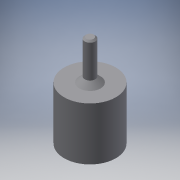
# Autodesk Inventor part: Transmission_Mount_Tester
Saved by Autodesk Inventor 2016 (Build 200138000, 138)
## iProperties
Created: 2015-07-24
Part Number: Transmission_Mount_Tester
Material: Generic
Document SubType Name: Modeling
Designer: 3DPrinterUser
Density: 1 g/cm^3
Appearance: Default
Author: 3DPrinterUser
Autodesk Inventor part; units mm, degrees
ref_plane "YZ Plane" through (0, 0, 0) normal (1, 0, 0) x (0, 1, 0)
ref_plane "XZ Plane" through (0, 0, 0) normal (0, 1, 0) x (-1, 0, 0)
ref_plane "XY Plane" through (0, 0, 0) normal (0, 0, 1) x (1, 0, 0)
sketch "Sketch1" plane through (0, 0, 0) normal (0, 0, 1) x (1, 0, 0)
  circle A0 centre (54.61, 0) radius 7.395 projected
  circle A1 centre (54.61, 0) radius 9.795
  point P0 (0, 0)
  dimension "d0" = 2.4
  constraints: 1 centre point, 1 coincident
  measures "d0" radial gap between concentric circles of A1 A0
extrude "Extrusion1" add sketch "Sketch1" against normal blind 20
sketch "Sketch2" plane through (54.61, 0, 0) normal (0, 0, 1) x (1, 0, 0)
  circle A0 centre (0, 0) radius 7.395 projected
  circle A1 centre (0, 0) radius 9.795 projected
  circle A2 centre (0, 0) radius 2 projected
  point P0 (-54.61, 0)
extrude "Extrusion2" add sketch "Sketch2" against normal blind 3 contours A0 | A1 | A2
sketch "Sketch3" plane through (54.61, 0, 0) normal (0, 0, 1) x (1, 0, 0)
  circle A0 centre (0, 0) radius 2 projected
  point P0 (-54.61, 0)
extrude "Extrusion3" add sketch "Sketch3" along normal blind 15
chamfer "Chamfer1" distance 2 angle 45 1 edges at (52.61, 0, 0)
chamfer "Chamfer2" distance 0.6 angle 45 1 edges at (52.61, 0, 15)
chamfer "Chamfer3" distance 7.39 angle 45 1 edges at (47.215, 0, -3)
body "Solid1"
